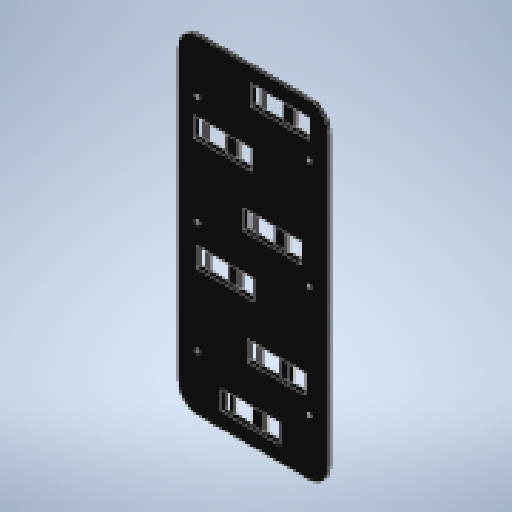
# Autodesk Inventor part: backplate-0
Saved by Autodesk Inventor 2023 (Build 270158030, 158C)
## iProperties
Created: 2024-09-24
Part Number: backplate-0
Material: Generic
Document SubType Name: Modeling
Designer: Imogen Heard
Density: 1 g/cm^3
Appearance: Glossy - Black
Author: Imogen Heard
Autodesk Inventor part; units mm, degrees
ref_plane "YZ Plane" through (0, 0, 0) normal (1, 0, 0) x (0, 1, 0)
ref_plane "XZ Plane" through (0, 0, 0) normal (0, 1, 0) x (-1, 0, 0)
ref_plane "XY Plane" through (0, 0, 0) normal (0, 0, 1) x (1, 0, 0)
ref_plane "Work Plane1" through (2.7698, 1, -3.5) normal (0, 0, 1) x (1, 0, 0)
sketch "Sketch1" plane through (0, 0, 0) normal (0, 0, 1) x (1, 0, 0)
  line L0 (34.0626, 1) -> (16.6619, 1) projected
  line L1 (34.0626, 14) -> (34.0626, 1) projected
  line L2 (16.6619, 14) -> (34.0626, 14) projected
  line L3 (16.6619, 14) -> (34.0626, 14) projected
  line L4 (34.0626, 15) -> (34.0626, 14) projected
  line L5 (34.0626, 15) -> (18.303, 15) projected
  line L6 (18.303, 0) -> (34.0626, 0) projected
  line L7 (18.303, 0) -> (34.0626, 0) projected
  line L8 (34.0626, 0) -> (34.0626, 1) projected
  line L9 (34.0626, 1) -> (16.6619, 1) projected
  line L10 (-15, 17) -> (56.6619, 17)
  line L11 (56.6619, 17) -> (56.6619, -2)
  line L12 (56.6619, -2) -> (-15, -2)
  line L13 (-15, -2) -> (-15, 17)
  line L14 (70.331, 1) -> (64.4317, 1) projected
  arc A0 (70.331, 1) -> (70.331, 14) centre (70.331, 7.5) ccw projected
  line L15 (64.4317, 14) -> (70.331, 14) projected
  line L16 (64.4317, 1) -> (64.4317, 14) projected
  arc A1 (70.331, 0) -> (70.331, 15) centre (70.331, 7.5) ccw projected
  line L17 (-22.7698, 1) -> (-28.669, 1) projected
  line L18 (-22.7698, 14) -> (-22.7698, 1) projected
  line L19 (-28.669, 14) -> (-22.7698, 14) projected
  arc A2 (-28.669, 14) -> (-28.669, 1) centre (-28.669, 7.5) ccw projected
  arc A3 (-28.669, 15) -> (-28.669, 0) centre (-28.669, 7.5) ccw projected
  line L20 (34.0626, 1) -> (41.6619, 1) projected
  line L21 (41.6619, 14) -> (34.0626, 14) projected
  line L22 (34.0626, 15) -> (41.004, 15) projected
  line L23 (41.004, 0) -> (34.0626, 0) projected
  line L24 (41.6619, 1) -> (41.6619, 14) projected
  line L25 (34.0626, 15) -> (39.0626, 15)
  line L26 (39.0626, 15) -> (39.0626, 0)
  line L27 (39.0626, 0) -> (34.0626, 0)
  line L28 (34.0626, 0) -> (34.0626, 15)
  arc A4 (18.303, 15) -> (16.6619, 14) centre (22.6619, 6) ccw projected
  line L29 (16.6619, 1) -> (16.6619, 14) projected
  arc A5 (16.6619, 1) -> (18.303, 0) centre (22.6619, 9) ccw projected
  line L30 (17.5119, 11.5) -> (18.2119, 11.5) projected
  line L31 (18.2119, 11.5) -> (18.2119, 3.5) projected
  line L32 (18.2119, 3.5) -> (17.5119, 3.5) projected
  line L33 (17.5119, 3.5) -> (17.5119, 11.5) projected
  line L34 (41.6619, 1) -> (5.1619, 1)
  line L35 (5.1619, 1) -> (5.1619, 14)
  line L36 (5.1619, 14) -> (41.6619, 14)
  line L37 (41.6619, 14) -> (41.6619, 1)
  line L38 (41.6619, 15) -> (5.1619, 15)
  line L39 (5.1619, 15) -> (5.1619, 0)
  line L40 (5.1619, 0) -> (41.6619, 0)
  line L41 (41.6619, 0) -> (41.6619, 15)
  point P0 (0, 0)
  point P1 (20.831, 17)
  point P2 (-30.669, 13.6847)
  point P3 (-30.669, 1.3153)
  point P4 (39.0626, 14)
  point P5 (39.0626, 1)
  point P6 (39.0626, 0)
  point P7 (16.6619, 14)
  point P8 (5.1619, 1)
  point P9 (5.1619, 14)
  dimension "d0" = 2
  dimension "d11" = 5
  dimension "d37" = 2
  dimension "d38" = 15
  dimension "d126" = 36.5
  constraints: 32 end point, 8 parallel, 4 horizontal, 4 perpendicular, 3 horizontal alignment, 2 vertical alignment, 1 midpoint
  measures "d0" distance from line of point (20.831, 17) L5
  measures "d11" distance between parallel lines of L26 L8
  measures "d37" distance between parallel lines of L12 L6
  measures "d38" distance between parallel lines of L24 L11
  measures "d126" distance between parallel lines of L35 L24
extrude "Extrusion1" add sketch "Sketch1" against normal up to surface (3.5 mm away) contours L10 L11 L12 L13
sketch "Sketch2" plane through (5.1411, 0, 0) normal (0, 1, 0) x (1, 0, 0)
  arc A0 (28.9215, 0) -> (36.5208, 3.5) centre (28.9215, 10) ccw projected
  line L0 (-2.3713, 3.5) -> (0.5208, 3.5) projected
  line L1 (30.0208, 2) -> (4.3589, 2)
  line L2 (13.5208, 3.5) -> (25.0208, 3.5)
  line L3 (25.0208, 3.5) -> (25.0208, 2.2)
  line L4 (25.0208, 2.2) -> (13.5208, 2.2)
  line L5 (13.5208, 2.2) -> (13.5208, 3.5)
  line L6 (26.5208, 3.5) -> (26.5208, 2)
  line L7 (10.5208, 2.2) -> (5.5208, 2.2)
  line L8 (5.5208, 2.2) -> (5.5208, 3.5)
  line L9 (5.5208, 3.5) -> (10.5208, 3.5)
  line L10 (10.5208, 3.5) -> (10.5208, 2.2)
  line L11 (0.0208, 3.5) -> (36.5208, 3.5) projected
  point P0 (12.0208, 3.5)
  point P1 (5.0208, 3.5)
  point P2 (6.0208, 3.5)
  point P3 (36.5208, 0)
  dimension "d6" = 1.5
  dimension "d7" = 0.2
  dimension "d117" = 11.5
  dimension "d118" = 3
  dimension "d119" = 5
  dimension "d127" = 1.5
  dimension "d128" = 10
  constraints: 18 end point, 4 horizontal alignment, 4 parallel, 2 horizontal, 2 perpendicular, 5 other
  measures "d7" distance between parallel lines of L1 L4
  measures "d117" distance between parallel lines of L5 L3
  measures "d118" distance between parallel lines of L10 L5
  measures "d119" distance between parallel lines of L8 L10
extrude "Extrusion2" add sketch "Sketch2" along normal up to surface (15 mm away)
sketch "Sketch11" plane through (0, 0, 0) normal (0, 0, 1) x (1, 0, 0)
  line L0 (5.1619, 0) -> (-2.6381, 0)
  line L1 (-2.6381, 0) -> (-2.6381, 15)
  line L2 (-2.6381, 15) -> (5.1619, 15)
  line L3 (5.1619, 15) -> (5.1619, 0)
  point P0 (0, 0)
  dimension "d120" = 7.8
  constraints: 8 end point, 3 coincident, 2 parallel, 1 horizontal, 1 perpendicular
  measures "d120" distance between parallel lines of L1 L3
extrude "Extrusion8" cut sketch "Sketch11" against normal blind 2.5
sketch "Sketch12" plane through (0, 0, -2.5) normal (0, 0, 1) x (1, 0, 0)
  line L0 (-2.6381, 15) -> (5.1619, 15) projected
  line L1 (-2.6381, 0) -> (-2.6381, 15) projected
  line L2 (5.1619, 0) -> (-2.6381, 0) projected
  line L3 (0.8619, 0) -> (-2.6381, 0)
  line L4 (-2.6381, 0) -> (-2.6381, 15)
  line L5 (-2.6381, 15) -> (0.8619, 15)
  line L6 (0.8619, 15) -> (0.8619, 0)
  line L7 (5.1619, 15) -> (5.1619, 0) projected
  point P0 (0, 0)
  point P1 (1.6411, 0)
  point P2 (0.8619, 0)
  dimension "d123" = 3.5
  constraints: 8 end point, 2 parallel, 1 horizontal, 1 perpendicular
  measures "d123" distance between parallel lines of L1 L6
extrude "Extrusion9" cut sketch "Sketch12" against normal through all contours L0 L6 L2 L1
chamfer "Chamfer1" distance 3.5 angle 45 1 edges at (41.6619, 7.5, -3.5)
chamfer "Chamfer4" distance 1 angle 45 1 edges at (30.1619, 7.5, -2.2)
chamfer "Chamfer5" distance 1 angle 45 1 edges at (29.1619, 7.5, -2.2)
chamfer "Chamfer6" distance 1 angle 45 1 edges at (28.1619, 7.5, -2.2)
sketch "Sketch6" plane through (0, 0, 0) normal (0, 0, 1) x (1, 0, 0)
  line L0 (-15, -2) -> (56.6619, -2) projected
  line L1 (56.6619, -2) -> (56.6619, 17) projected
  line L2 (56.6619, 17) -> (-15, 17) projected
  line L3 (-15, 17) -> (-15, -2) projected
  line L4 (-2.6381, 0) -> (-2.6381, 15) projected
  line L5 (-2.6381, 15) -> (41.6619, 15) projected
  line L6 (41.6619, 0) -> (-2.6381, 0) projected
  line L7 (41.6619, 15) -> (41.6619, 0) projected
  point P0 (0, 0)
extrude "Extrusion5" add sketch "Sketch6" along normal blind 0.5
sketch "Sketch13" plane through (10.6619, 0, -2.2) normal (0, 0, 1) x (1, 0, 0)
  line L0 (0, 15) -> (5, 15) projected
  line L1 (0, 0) -> (0, 15) projected
  line L2 (5, 0) -> (0, 0) projected
  line L3 (5, 0) -> (5, 15) projected
  point P0 (-10.6619, 0)
extrude "Extrusion10" cut sketch "Sketch13" against normal through all
chamfer "Chamfer9" distance 1 angle 45 1 edges at (5.1619, 7.5, -2.5)
pattern_linear "Rectangular Pattern1" [suppressed]
sketch "Sketch7" plane through (0, 0, 0.5) normal (0, 0, 1) x (1, 0, 0)
  line L0 (56.6619, -2) -> (56.6619, 17) projected
  line L1 (56.6619, -2) -> (56.6619, 17) projected
  line L2 (56.6619, 17) -> (-15, 17) projected
  line L3 (-15, 17) -> (-15, -2) projected
  line L4 (-15, -2) -> (56.6619, -2) projected
  line L5 (79.8562, 232) -> (8.1943, 232)
  line L6 (8.1943, 232) -> (8.1943, 213)
  line L7 (8.1943, 213) -> (79.8562, 213)
  line L8 (79.8562, 213) -> (79.8562, 232)
  line L9 (35.5797, 189) -> (-36.0822, 189)
  line L10 (-36.0822, 189) -> (-36.0822, 170)
  line L11 (-36.0822, 170) -> (35.5797, 170)
  line L12 (35.5797, 170) -> (35.5797, 189)
  line L13 (1.7035, 146) -> (1.7035, 127)
  line L14 (73.3654, 146) -> (1.7035, 146)
  line L15 (1.7035, 127) -> (73.3654, 127)
  line L16 (73.3654, 127) -> (73.3654, 146)
  line L17 (5.3123, 60) -> (5.3123, 41)
  line L18 (76.9742, 60) -> (5.3123, 60)
  line L19 (5.3123, 41) -> (76.9742, 41)
  line L20 (76.9742, 41) -> (76.9742, 60)
  line L21 (-34.2741, 103) -> (-34.2741, 84)
  line L22 (37.3878, 84) -> (37.3878, 103)
  line L23 (-34.2741, 84) -> (37.3878, 84)
  line L24 (37.3878, 103) -> (-34.2741, 103)
  point P0 (0, 0)
  point P1 (37.5345, 146)
  point P2 (44.0253, 232)
  dimension "d55" = 19
  dimension "d56" = 71.6619
  dimension "d57" = 71.6619
  dimension "d58" = 19
  dimension "d61" = 71.6619
  dimension "d62" = 19
  dimension "d65" = 71.6619
  dimension "d66" = 19
  dimension "d71" = 71.6619
  dimension "d72" = 19
  dimension "d73" = 71.6619
  dimension "d74" = 19
  dimension "d81" = 43
  dimension "d82" = 43
  dimension "d83" = 43
  dimension "d84" = 43
  dimension "d88" = 43
  dimension "d89" = 234
  constraints: 40 end point, 10 parallel, 5 coincident, 5 horizontal, 5 perpendicular, 2 midpoint
  measures "d55" distance between parallel lines of L4 L2
  measures "d56" distance between parallel lines of L3 L1
  measures "d57" distance between parallel lines of L6 L8
  measures "d58" distance between parallel lines of L7 L5
  measures "d61" distance between parallel lines of L10 L12
  measures "d62" distance between parallel lines of L11 L9
  measures "d65" distance between parallel lines of L13 L16
  measures "d66" distance between parallel lines of L15 L14
  measures "d71" distance between parallel lines of L17 L20
  measures "d72" distance between parallel lines of L19 L18
  measures "d73" distance between parallel lines of L21 L22
  measures "d74" distance between parallel lines of L23 L24
  measures "d81" distance between parallel lines of L9 L5
  measures "d82" distance between parallel lines of L14 L9
  measures "d83" distance from line of L24 point (37.534, 146)
  measures "d84" distance between parallel lines of L18 L24
  measures "d88" distance between parallel lines of L19 L4
  measures "d89" distance from line of point (44.025, 232) L4
pattern_sketch "Sketch Driven Pattern1" from (56.6619, 17, 0.5) copies at (79.8562, 232, 0.5) at (35.5797, 189, 0.5) at (73.3654, 146, 0.5) at (37.3878, 103, 0.5) at (76.9742, 60, 0.5)
sketch "Sketch8" plane through (0, 0, 0.5) normal (0, 0, 1) x (1, 0, 0)
  line L0 (-36.0822, -2) -> (79.8562, -2)
  line L1 (79.8562, -2) -> (79.8562, 232)
  line L2 (79.8562, 232) -> (-36.0822, 232)
  line L3 (-36.0822, 232) -> (-36.0822, -2)
  line L4 (56.6619, -2) -> (56.6619, 17) projected
  line L5 (56.6619, 17) -> (-15, 17) projected
  line L6 (-15, 17) -> (-15, -2) projected
  line L7 (-15, -2) -> (56.6619, -2) projected
  line L8 (76.9742, 41) -> (76.9742, 60) projected
  line L9 (76.9742, 60) -> (5.3123, 60) projected
  line L10 (5.3123, 60) -> (5.3123, 41) projected
  line L11 (5.3123, 41) -> (76.9742, 41) projected
  line L12 (37.3878, 84) -> (37.3878, 103) projected
  line L13 (37.3878, 103) -> (-34.2741, 103) projected
  line L14 (-34.2741, 103) -> (-34.2741, 84) projected
  line L15 (-34.2741, 84) -> (37.3878, 84) projected
  line L16 (73.3654, 127) -> (73.3654, 146) projected
  line L17 (73.3654, 146) -> (1.7035, 146) projected
  line L18 (1.7035, 146) -> (1.7035, 127) projected
  line L19 (1.7035, 127) -> (73.3654, 127) projected
  line L20 (35.5797, 170) -> (35.5797, 189) projected
  line L21 (35.5797, 189) -> (-36.0822, 189) projected
  line L22 (-36.0822, 189) -> (-36.0822, 170) projected
  line L23 (-36.0822, 170) -> (35.5797, 170) projected
  line L24 (79.8562, 213) -> (79.8562, 232) projected
  line L25 (79.8562, 232) -> (8.1943, 232) projected
  line L26 (8.1943, 232) -> (8.1943, 213) projected
  line L27 (8.1943, 213) -> (79.8562, 213) projected
  line L28 (79.8562, -2) -> (-36.0822, -2)
  line L29 (-36.0822, -2) -> (-36.0822, -12)
  line L30 (-36.0822, -12) -> (79.8562, -12)
  line L31 (79.8562, -12) -> (79.8562, -2)
  line L32 (79.8562, 213) -> (79.8562, 232) projected
  line L33 (79.8562, 232) -> (-36.0822, 232)
  line L34 (-36.0822, 232) -> (-36.0822, 242)
  line L35 (-36.0822, 242) -> (79.8562, 242)
  line L36 (79.8562, 242) -> (79.8562, 232)
  point P0 (0, 0)
  point P1 (8.1943, 232)
  point P2 (-36.0822, 189)
  point P3 (-36.0822, 170)
  point P4 (-36.0822, 232)
  dimension "d97" = 254
  dimension "d134" = 10
  dimension "d135" = 10
  constraints: 24 end point, 6 parallel, 3 horizontal, 3 perpendicular, 1 coincident, 1 horizontal alignment, 1 point on line, 1 vertical alignment
  measures "d97" distance between parallel lines of L35 L30
  measures "d134" distance between parallel lines of L30 L0
  measures "d135" distance between parallel lines of L35 L2
extrude "Extrusion6" add sketch "Sketch8" against normal up to surface (4 mm away) contours L3 L23 L20 L21 L2 L26 L27 L1 L0 L4 L5 L6 | L0 L31 L30 L29 | L34 L35 L36 L2
fillet "Fillet2" radius 15 4 edges at (-36.0822, -12, -1.5) (79.8562, -12, -1.5) (-36.0822, 242, -1.5) (79.8562, 242, -1.5)
chamfer "Chamfer7" distance 5 distance2 2 8 edges at (-31.6888, -7.6066, -3.5) (21.887, -12, -3.5) (75.4628, -7.6066, -3.5) (79.8562, 115, -3.5) (75.4628, 237.6066, -3.5) (21.887, 242, -3.5) (-31.6888, 237.6066, -3.5) (-36.0822, 115, -3.5) measured on face at (21.887, -11.5, -3.5) measured on face at (-31.3353, -7.253, -3.5) measured on face at (75.1093, 237.253, -3.5) measured on face at (79.3562, 115, -3.5) measured on face at (-31.3353, 237.253, -3.5) measured on face at (75.1093, -7.253, -3.5) measured on face at (-35.5822, 115, -3.5) measured on face at (21.887, 241.5, -3.5)
sketch "Sketch9" plane through (64.8562, 237, -3.5) normal (0, 0, -1) x (-1, 0, 0)
  circle A0 centre (0, -206) radius 1.55
  circle A1 centre (85.9385, -206) radius 1.55
  circle A2 centre (85.9385, -36) radius 1.55
  circle A3 centre (0, -36) radius 1.55
  line L0 (-15, -10) -> (-15, -234) projected
  line L1 (100.9385, -234) -> (100.9385, -10) projected
  line L2 (19.6943, -222) -> (34.6943, -222) projected
  line L3 (14.382, -194) -> (25.882, -194) projected
  line L4 (0, -249) -> (85.9385, -249) projected
  line L5 (85.9385, 5) -> (0, 5) projected
  line L6 (40.7766, -50) -> (55.7766, -50) projected
  line L7 (11.5, -22) -> (23, -22) projected
  circle A4 centre (0, -120) radius 1.55
  circle A5 centre (85.9385, -120) radius 1.55
  line L8 (38.9685, -136) -> (53.9685, -136) projected
  line L9 (17.9908, -108) -> (29.4908, -108) projected
  point P0 (64.8562, -237)
  point P1 (22.2937, -240)
  point P2 (1.9813, -208)
  point P3 (43.3759, -52)
  point P4 (-0.9007, -20)
  point P5 (41.5678, -146)
  point P6 (43.7361, -136)
  point P7 (5.5902, -114)
  dimension "d101" = 3.1
  dimension "d102" = 15
  dimension "d103" = 15
  dimension "d104" = 16
  dimension "d105" = 12
  dimension "d106" = 43
  dimension "d107" = 41
  dimension "d108" = 14
  dimension "d109" = 14
  dimension "d110" = 16
  dimension "d111" = 12
  constraints: 6 centre point, 5 equal radius, 4 vertical alignment, 3 horizontal alignment, 7 other
  measures "d101" diameter of A0
  measures "d102" distance from line of L0 A0.centre
  measures "d103" distance from line of L1 A1.centre
  measures "d106" distance from line of L4 A0.centre
  measures "d107" distance from line of L5 A3.centre
  measures "d110" vertical distance of A4.centre point (43.736, -136)
extrude "Extrusion7" cut sketch "Sketch9" against normal through all
chamfer "Chamfer8" distance 3 angle 45 6 edges at (-19.5322, 201, -3.5) (66.4062, 201, -3.5) (66.4062, 117, -3.5) (-19.5322, 117, -3.5) (-19.5322, 31, -3.5) (66.4062, 31, -3.5)
equation "\"d57\" = d56"
equation "\"d58\" = d55"
equation "\"d61\" = d63"
equation "\"d62\" = d64"
equation "\"d65\" = d67"
equation "\"d66\" = d68"
equation "\"d71\" = d77"
equation "\"d72\" = d78"
equation "\"d73\" = d79"
equation "\"d74\" = d80"
equation "\"d81\" = d88"
equation "\"d82\" = d88"
equation "\"d83\" = d88"
equation "\"d84\" = d88"
equation "\"d63\" = 71.661904"
equation "\"d64\" = 19"
equation "\"d67\" = 71.661904"
equation "\"d68\" = 19"
equation "\"d77\" = 71.661904"
equation "\"d78\" = 19"
equation "\"d79\" = 71.661904"
equation "\"d80\" = 19"
